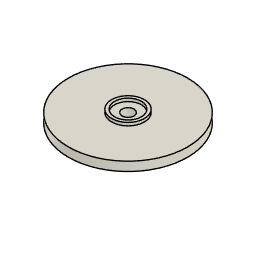
Savöx_SH_0255 MG_micro_servo_horn (Autodesk Fusion 360 design; units mm, degrees)
Autodesk Fusion 360 part; units mm, degrees
sketch "Horn Body" plane through (0, 0, 0) normal (0, 0, 1) x (1, 0, 0)
  circle A0 centre (0, 0) radius 10
  dimension "d1" = 20
  constraint coincident A0.centre origin
  measures "d1" diameter of A0
extrude "Extrude1" add sketch "Horn Body" along normal blind 1.5
sketch "Connector" plane through (0, 0, 0) normal (0, 0, -1) x (1, 0, 0)
  circle A0 centre (0, 0) radius 10
  circle A1 centre (0, 0) radius 2.5
  circle A2 centre (0, 0) radius 3.5
  dimension "d4" = 5
  dimension "d5" = 7
  constraint concentric A0 A1
  constraint concentric A1 A2
  measures "d4" diameter of A1
  measures "d5" diameter of A2
extrude "Extrude2" add sketch "Connector" along normal blind 3.5 contours A2
sketch "Screw Hole" plane through (0, 0, 1.5) normal (0, 0, 1) x (-1, 0, 0)
  circle A0 centre (0, 0) radius 10
  circle A1 centre (0, 0) radius 2.75
  circle A2 centre (0, 0) radius 2.25
  circle A3 centre (0, 0) radius 1
  dimension "d8" = 5.5
  dimension "d9" = 4.5
  dimension "d10" = 2
  constraint coincident A0.centre A1.centre
  constraint concentric A2 A3
  measures "d8" diameter of A1
  measures "d9" diameter of A2
  measures "d10" diameter of A3
extrude "Extrude3" add sketch "Screw Hole" along normal blind 0.5 contours A1
extrude "Extrude4" cut sketch "Screw Hole" against normal blind 1.5 contours A3
named bodies: "Savöx SH 0255 MG Micro Servo Horn"
